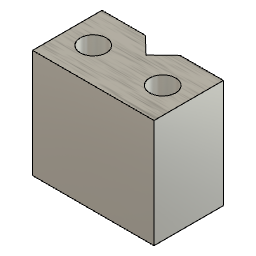
Solution 2 (Autodesk Fusion 360 design; units mm, degrees)
Autodesk Fusion 360 part; units mm, degrees
sketch "Sketch3" plane through (0, 0, 0) normal (0, 1, 0) x (1, 0, 0)
  line L0 (0, 0) -> (0, -16)
  line L1 (28, 0) -> (28, -16)
  line L2 (0, -16) -> (28, -16)
  line L3 (14, -3.862) -> (10, 0)
  line L4 (14, -3.862) -> (18, 0)
  line L5 (0, 0) -> (10, 0)
  line L6 (18, 0) -> (28, 0)
  circle A0 centre (6, -8) radius 3
  circle A1 centre (22.0006, -8) radius 3
  dimension "d21" = 16
  dimension "d22" = 28
  dimension "d23" = 16
  dimension "d25" = 6
  dimension "d26" = 6
  constraint coincident L0.start L5.start
  constraint vertical L0
  constraint perpendicular L0 L5
  constraint perpendicular L1 L5
  constraint coincident L4.end L5
  constraint collinear L5 L6
  measures "d21" distance of L0.start L0.end
  measures "d22" distance of L0.start L1.start
  measures "d23" distance of L1.start L1.end
  measures "d25" diameter of A0
  measures "d26" diameter of A1
extrude "Extrude3" add sketch "Sketch3" along normal blind 5
extrude "Extrude4" add 1 faces at (11.6987, 5, 14.2642) along direction (0, 1, 0) blind 20
